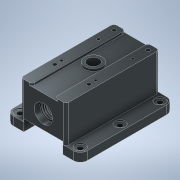
# Autodesk Inventor part: 1-夹具体
Saved by Autodesk Inventor 2022 (Build 260153000, 153)
## iProperties
Created: 2023-01-07
Part Number: 1-夹具体
Material: 灰口铁
Document SubType Name: Modeling
Designer: Lzy18
Density: 7.15 g/cm^3
Appearance: 灰口铁
Author: Lzy18
Autodesk Inventor part; units mm, degrees
ref_plane "YZ Plane" through (0, 0, 0) normal (1, 0, 0) x (0, 1, 0)
ref_plane "XZ Plane" through (0, 0, 0) normal (0, 1, 0) x (-1, 0, 0)
ref_plane "XY Plane" through (0, 0, 0) normal (0, 0, 1) x (1, 0, 0)
sketch "草图1" plane through (0, 0, 0) normal (0, 1, 0) x (-1, 0, 0)
  line L0 (65, 82) -> (-65, 82)
  line L1 (-65, 82) -> (-65, -82)
  line L2 (-65, -82) -> (65, -82)
  line L3 (65, -82) -> (65, 82)
  line L4 (65, 82) -> (-65, -82) construction
  line L5 (-65, 82) -> (65, -82) construction
  point P0 (0, 0)
  dimension "d0" = 130
  dimension "d1" = 164
  constraints: 12 end point, 2 midpoint, 2 parallel, 1 horizontal, 1 perpendicular
  measures "d0" distance of L2.end L1.end
  measures "d1" distance of L1.end L0.end
extrude "拉伸1" add sketch "草图1" along normal blind 15
sketch "草图2" plane through (0, 15, 0) normal (0, 1, 0) x (1, 0, 0)
  line L0 (-40, -82) -> (40, -82)
  line L1 (40, -82) -> (40, 82)
  line L2 (40, 82) -> (-40, 82)
  line L3 (-40, 82) -> (-40, -82)
  line L4 (-40, -82) -> (40, 82) construction
  line L5 (40, -82) -> (-40, 82) construction
  point P0 (0, 0)
  dimension "d4" = 80
  dimension "d5" = 164
  constraints: 12 end point, 2 midpoint, 2 parallel, 1 horizontal, 1 perpendicular
  measures "d4" distance of L2.end L1.end
  measures "d5" distance of L1.end L0.end
extrude "拉伸2" add sketch "草图2" along normal blind 65
sketch "草图3" plane through (0, 0, 0) normal (0, -1, 0) x (1, 0, 0)
  line L0 (34.5, 82) -> (-34.5, 82)
  line L1 (-34.5, 82) -> (-34.5, -82)
  line L2 (-34.5, -82) -> (34.5, -82)
  line L3 (34.5, -82) -> (34.5, 82)
  line L4 (34.5, 82) -> (-34.5, -82) construction
  line L5 (-34.5, 82) -> (34.5, -82) construction
  point P0 (0, 0)
  dimension "d8" = 69
  dimension "d9" = 164
  constraints: 12 end point, 2 midpoint, 2 parallel, 1 horizontal, 1 perpendicular
  measures "d8" distance of L2.end L1.end
  measures "d9" distance of L1.end L0.end
extrude "拉伸3" cut sketch "草图3" against normal blind 20
sketch "草图10" plane through (0, 80, 0) normal (0, 1, 0) x (1, 0, 0)
  line L0 (40, -82) -> (40, 82) projected
  line L1 (40, 82) -> (-40, 82) projected
  line L2 (-40, 82) -> (-40, -82) projected
  line L3 (-40, -82) -> (40, -82) projected
  arc A0 (10, 6) -> (-10, 6) centre (0, 6) ccw projected
  circle A1 centre (0, 6) radius 15
  line L4 (40, 82) -> (-40, 82) projected
  line L5 (-20, 82) -> (-20, -82)
  line L6 (-34.5, -82) -> (34.5, -82) projected
  line L7 (20, 82) -> (20, -82)
  line L8 (-40, -82) -> (40, -82) projected
  point P0 (0, 0)
  dimension "d66" = 30
  dimension "d67" = 20
  dimension "d68" = 20
  constraints: 4 end point, 4 point on line, 2 perpendicular, 1 centre point, 1 coincident
  measures "d66" diameter of A1
  measures "d67" distance between parallel lines of L2 L5
  measures "d68" distance between parallel lines of L0 L7
extrude "拉伸4" cut sketch "草图10" against normal blind 4 contours L7 L3 L5 L1
sketch "草图28" plane through (0, 80, -6) normal (0, 1, 0) x (1, 0, 0)
  circle A0 centre (0, 0) radius 15 projected
  point P0 (0, -6)
  constraints: 1 coincident
hole "孔19" at (0, 80, -6) direction (0, -1, 0) diameter 20 depth 25
sketch "草图39" plane through (0, 80, 0) normal (0, 1, 0) x (1, 0, 0)
  line L0 (0, -4) -> (0, 16) projected
  line L1 (40, 82) -> (20, 82) projected
  circle A0 centre (30, 45) radius 2.5
  circle A1 centre (30, -20) radius 2.5
  point P0 (0, 0)
  dimension "d287" = 5
  dimension "d289" = 5
  dimension "d290" = 65
  constraints: 2 centre point
  measures "d287" diameter of A0
  measures "d289" diameter of A1
  measures "d290" distance of A1.centre A0.centre
extrude "拉伸9" cut sketch "草图39" against normal blind 20
sketch "草图40" plane through (0, 80, 0) normal (0, 1, 0) x (1, 0, 0)
  circle A0 centre (30, 45) radius 2.5 projected
  circle A1 centre (30, 72) radius 4
  point P0 (0, 0)
  dimension "d295" = 8
  dimension "d296" = 27
  constraints: 1 centre point
  measures "d295" diameter of A1
  measures "d296" distance of A0.centre A1.centre
hole "孔26" at (30, 80, -72) direction (0, -1, 0) diameter 6.647 depth 25 thread size "M8x1.25" designation "M8" class "6H" standard "GB Metric profile"
sketch "草图41" plane through (0, 80, 0) normal (0, 1, 0) x (1, 0, 0)
  circle A0 centre (30, -20) radius 2.5 projected
  point P0 (0, 0)
  point P1 (30, -32)
  dimension "d304" = 12
  measures "d304" distance of A0.centre point (30, -32)
hole "孔27" at (30, 80, 32) direction (0, -1, 0) diameter 6.647 depth 25 thread size "M8x1.25" designation "M8" class "6H" standard "GB Metric profile"
mirror "镜像10" about plane through (0, 0, 0) normal (1, 0, 0) of "孔26", "拉伸9", "孔27"
fillet "圆角3" radius 12 4 edges at (-65, 7.5, -82) (-65, 7.5, 82) (65, 7.5, 82) (65, 7.5, -82)
fillet "圆角4" radius 5 8 edges at (20, 78, 82) (20, 78, -82) (40, 47.5, -82) (40, 47.5, 82) (-40, 47.5, 82) (-40, 47.5, -82) (-20, 78, 82) (-20, 78, -82)
sketch "草图42" plane through (-34.5, 20, 82) normal (0, 0, 1) x (1, 0, 0)
  line L0 (69, -20) -> (87.5, -20) projected
  point P0 (34.5, -20)
  point P1 (34.5, 25)
  dimension "d314" = 45
  measures "d314" distance from line of L0 point (34.5, 25)
hole "孔28" at (0, 45, 82) direction (0, 0, -1) diameter 26.211 depth 29 counterbore diameter 32 counterbore depth 10 thread size "M30x3.5" designation "M30" class "6H" standard "GB Metric profile"
sketch "草图43" plane through (0, 45, 53) normal (0, 0, 1) x (1, 0, 0)
  circle A0 centre (0, 0) radius 13.1055 projected
  point P0 (0, -45)
  constraints: 1 coincident
hole "孔29" at (0, 45, 53) direction (0, 0, -1) diameter 20 depth 95 counterbore diameter 32 counterbore depth 7
sketch "草图44" plane through (0, 45, -42) normal (0, 0, 1) x (1, 0, 0)
  circle A0 centre (0, 0) radius 10 projected
  point P0 (0, -45)
  constraints: 2 coincident
hole "孔30" at (0, 45, -42) at (0, 45, -42) direction (0, 0, -1) diameter 20.752 end through all counterbore diameter 26 counterbore depth 7 thread size "M24x3" designation "M24" class "6H" standard "GB Metric profile"
sketch "草图45" plane through (0, 15, 0) normal (0, 1, 0) x (1, 0, 0)
  circle A0 centre (-53, 0) radius 9
  line L0 (0, 16) -> (0, -4) projected
  circle A1 centre (-53, -70) radius 9
  line L1 (-44, 0) -> (-62, 0)
  circle A2 centre (-53, 70) radius 9
  point P0 (0, 0)
  dimension "d336" = 18
  dimension "d337" = 53
  dimension "d338" = 18
  dimension "d339" = 70
  constraints: 3 centre point, 2 end point, 2 point on circle, 1 horizontal, 1 symmetric about line, 1 other
  measures "d336" diameter of A0
  measures "d337" distance from line of L0 A0.centre
  measures "d338" diameter of A1
  measures "d339" distance of A0.centre A1.centre
extrude "拉伸10" cut sketch "草图45" against normal blind 2
sketch "草图46" plane through (-53, 13, 70) normal (0, 1, 0) x (1, 0, 0)
  circle A0 centre (0, 0) radius 9 projected
  point P0 (53, 70)
  constraints: 1 coincident
hole "孔31" at (-53, 13, 70) direction (0, -1, 0) diameter 9 end through all
sketch "草图47" plane through (-53, 13, 0) normal (0, 1, 0) x (1, 0, 0)
  circle A0 centre (0, 0) radius 9 projected
  point P0 (53, 0)
  constraints: 1 coincident
hole "孔32" at (-53, 13, 0) direction (0, -1, 0) diameter 9 end through all
sketch "草图48" plane through (-53, 13, -70) normal (0, 1, 0) x (1, 0, 0)
  circle A0 centre (0, 0) radius 9 projected
  point P0 (53, -70)
  constraints: 1 coincident
hole "孔33" at (-53, 13, -70) direction (0, -1, 0) diameter 9 end through all
mirror "镜像11" about plane through (0, 0, 0) normal (1, 0, 0) of "拉伸10", "孔31", "孔32", "孔33"
